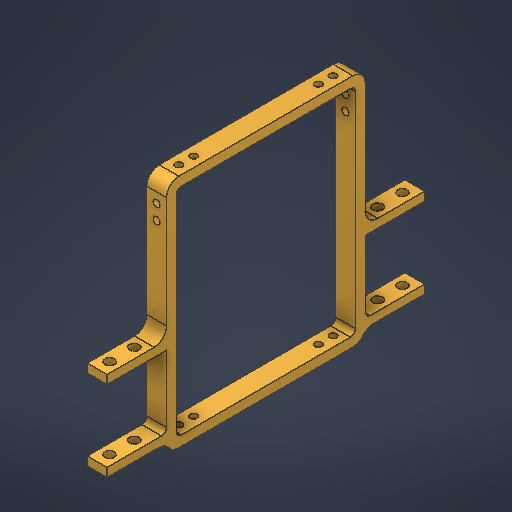
# Autodesk Inventor part: structural_ring1
Saved by Autodesk Inventor 2026.1 (Build 301233000, 233)
## iProperties
Created: 2026-05-16
Part Number: structural_ring1
Material: Generic
Document SubType Name: Modeling
Designer: emanuel
Density: 1 g/cm^3
Appearance: Default
Author: emanuel
Autodesk Inventor part; units mm, degrees
ref_plane "YZ Plane" through (0, 0, 0) normal (1, 0, 0) x (0, 1, 0)
ref_plane "XZ Plane" through (0, 0, 0) normal (0, 1, 0) x (-1, 0, 0)
ref_plane "XY Plane" through (0, 0, 0) normal (0, 0, 1) x (1, 0, 0)
sketch "Sketch1" plane through (0, 0, 0) normal (1, 0, 0) x (0, 1, 0)
  line L0 (0, 40.15) -> (0, -40.15)
  line L1 (-47.5, 0) -> (47.5, 0)
  line L2 (-47.5, 40.15) -> (47.5, 40.15)
  line L3 (47.5, 40.15) -> (47.5, -40.15)
  line L4 (47.5, -40.15) -> (-47.5, -40.15)
  line L5 (-47.5, -40.15) -> (-47.5, 40.15)
  line L6 (-47.5, 40.15) -> (47.5, -40.15) construction
  line L7 (47.5, 40.15) -> (-47.5, -40.15) construction
  line L8 (47.5, 40.15) -> (43.5, 40.15)
  line L9 (43.5, 40.15) -> (43.5, 36.15)
  line L10 (43.5, 36.15) -> (47.5, 36.15)
  line L11 (47.5, 36.15) -> (47.5, 40.15)
  line L12 (47.5, -40.15) -> (43.5, -40.15)
  line L13 (43.5, -40.15) -> (43.5, -36.15)
  line L14 (43.5, -36.15) -> (47.5, -36.15)
  line L15 (47.5, -36.15) -> (47.5, -40.15)
  line L16 (-47.5, -40.15) -> (-43.5, -40.15)
  line L17 (-43.5, -40.15) -> (-43.5, -36.15)
  line L18 (-43.5, -36.15) -> (-47.5, -36.15)
  line L19 (-47.5, -36.15) -> (-47.5, -40.15)
  line L20 (-43.5, -36.15) -> (43.5, -36.15)
  line L21 (43.5, -36.15) -> (43.5, 36.15)
  line L22 (43.5, 36.15) -> (-43.5, 36.15)
  line L23 (-43.5, 36.15) -> (-43.5, -36.15)
  point P0 (0, 0)
  dimension "d0" = 80.3
  dimension "d1" = 95
  dimension "d2" = 4
  dimension "d3" = 4
  dimension "d4" = 4
  dimension "d5" = 4
  dimension "d6" = 4
  dimension "d7" = 4
  dimension "d51" = 80.3
  constraints: 48 end point, 10 parallel, 6 horizontal, 5 perpendicular, 4 midpoint, 1 vertical
  measures "d0" distance of L0.start L0.end
  measures "d1" distance of L1.start L1.end
  measures "d2" distance of L10.end L9.end
  measures "d3" distance of L9.end L8.end
  measures "d4" distance of L13.end L14.end
  measures "d5" distance of L12.end L13.end
  measures "d6" distance of L18.end L17.end
  measures "d7" distance of L17.end L16.end
  measures "d51" distance between parallel lines of L4 L2
extrude "Extrusion1" add sketch "Sketch1" along normal blind 8 contours L2 L9 L22 L0 | L0 L22 L23 L1 L5 L2 | L2 L3 L10 L9 | L10 L3 L1 L21 | L1 L23 L18 L5 | L20 L13 L4 L0 | L0 L4 L17 L20 | L1 L3 L14 L21 | L18 L17 L4 L5 | L14 L3 L4 L13
sketch "Sketch2" plane through (8, 0, 0) normal (1, 0, 0) x (0, 0, -1)
  line L0 (40.15, 47.5) -> (-40.15, 47.5) projected
  line L1 (40.15, 47.5) -> (40.15, -10.9)
  line L2 (40.15, -47.5) -> (40.15, 47.5) projected
  line L3 (40.15, -10.9) -> (64.15, -10.9)
  line L4 (64.15, -10.9) -> (64.15, -7.4)
  line L5 (64.15, -7.4) -> (40.15, -7.4)
  line L6 (40.15, -7.4) -> (40.15, -10.9)
  line L7 (40.15, -10.9) -> (40.15, -39.9)
  line L8 (40.15, -39.9) -> (64.15, -39.9)
  line L9 (64.15, -39.9) -> (64.15, -43.4)
  line L10 (64.15, -43.4) -> (40.15, -43.4)
  line L11 (40.15, -43.4) -> (40.15, -39.9)
  line L12 (0, 47.5) -> (0, 43.5)
  line L13 (-36.15, 43.5) -> (36.15, 43.5) projected
  line L14 (-40.15, 47.5) -> (-40.15, -10.9)
  line L15 (-40.15, -47.5) -> (-40.15, 47.5)
  line L16 (-40.15, -10.9) -> (-64.15, -10.9)
  line L17 (-64.15, -10.9) -> (-64.15, -7.4)
  line L18 (-64.15, -7.4) -> (-40.15, -7.4)
  line L19 (-40.15, -7.4) -> (-40.15, -10.9)
  line L20 (-40.15, -10.9) -> (-40.15, -39.9)
  line L21 (-40.15, -39.9) -> (-64.15, -39.9)
  line L22 (-64.15, -39.9) -> (-64.15, -43.4)
  line L23 (-64.15, -43.4) -> (-40.15, -43.4)
  line L24 (-40.15, -43.4) -> (-40.15, -39.9)
  point P0 (0, 0)
  dimension "d10" = 58.4
  dimension "d11" = 24
  dimension "d12" = 3.5
  dimension "d13" = 29
  dimension "d14" = 24
  dimension "d15" = 3.5
  constraints: 44 end point, 9 symmetric about line, 4 parallel, 4 point on line, 2 horizontal, 2 midpoint, 2 perpendicular
  measures "d10" distance of L0.start L1.end
  measures "d11" distance of L5.end L4.end
  measures "d12" distance of L4.end L3.end
  measures "d13" distance of L1.end L7.end
  measures "d14" distance of L9.end L10.end
  measures "d15" distance of L8.end L9.end
extrude "Extrusion2" add sketch "Sketch2" against normal blind 8
sketch "Sketch3" plane through (8, -7.4, 64.15) normal (0, 1, 0) x (1, 0, 0)
  line L0 (0, 0) -> (-8, 0) projected
  line L1 (-4, 0) -> (-4, 5)
  line L2 (-4, 5) -> (-4, 15)
  circle A0 centre (-4, 5) radius 2
  circle A1 centre (-4, 15) radius 2
  line L3 (0, 128.3) -> (-8, 128.3) projected
  line L4 (-4, 128.3) -> (-4, 123.3)
  line L5 (-4, 123.3) -> (-4, 113.3)
  circle A2 centre (-4, 113.3) radius 2
  circle A3 centre (-4, 123.3) radius 2
  point P0 (-8, 64.15)
  dimension "d18" = 5
  dimension "d19" = 10
  dimension "d20" = 4
  dimension "d21" = 4
  dimension "d22" = 5
  dimension "d23" = 10
  dimension "d24" = 4
  dimension "d25" = 4
  constraints: 8 end point, 4 centre point, 4 coincident, 2 midpoint, 2 point on line, 2 vertical
  measures "d18" distance of L1.start L1.end
  measures "d19" distance of L1.end L2.end
  measures "d20" diameter of A0
  measures "d21" diameter of A1
  measures "d22" distance of L4.start L4.end
  measures "d23" distance of L4.end L5.end
  measures "d24" diameter of A2
  measures "d25" diameter of A3
extrude "Extrusion3" cut sketch "Sketch3" against normal blind 50
fillet "Fillet1" radius 5 4 edges at (4, 47.5, 40.15) (4, 47.5, -40.15) (4, -47.5, 40.15) (4, -47.5, -40.15)
fillet "Fillet2" radius 2 4 edges at (4, -43.5, -36.15) (4, -43.5, 36.15) (4, 43.5, 36.15) (4, 43.5, -36.15)
sketch "Sketch4" plane through (0, 47.5, 35.15) normal (0, 1, 0) x (1, 0, 0)
  line L0 (8, 0) -> (0, 0) projected
  line L1 (8, 0) -> (4, 0)
  line L2 (4, 0) -> (4, 4)
  line L3 (4, 4) -> (8, 4)
  line L4 (8, 4) -> (8, 0)
  line L5 (0, 70.3) -> (8, 70.3) projected
  line L6 (0, 70.3) -> (4, 70.3)
  line L7 (4, 70.3) -> (4, 66.3)
  line L8 (4, 66.3) -> (0, 66.3)
  line L9 (0, 66.3) -> (0, 70.3)
  line L10 (4, 66.3) -> (4, 60.3)
  line L11 (4, 4) -> (4, 10)
  circle A0 centre (4, 66.3) radius 1.45
  circle A1 centre (4, 60.3) radius 1.45
  circle A2 centre (4, 10) radius 1.45
  circle A3 centre (4, 4) radius 1.45
  point P0 (0, 35.15)
  dimension "d30" = 4
  dimension "d31" = 4
  dimension "d32" = 4
  dimension "d33" = 4
  dimension "d34" = 6
  dimension "d35" = 6
  dimension "d36" = 2.9
  dimension "d37" = 2.9
  dimension "d38" = 2.9
  dimension "d39" = 2.9
  constraints: 20 end point, 4 centre point, 4 coincident, 4 parallel, 2 horizontal, 2 perpendicular, 2 vertical
  measures "d30" distance of L2.end L3.end
  measures "d31" distance of L1.end L2.end
  measures "d32" distance of L7.end L8.end
  measures "d33" distance of L6.end L7.end
  measures "d34" distance of L7.end L10.end
  measures "d35" distance of L2.end L11.end
  measures "d36" diameter of A0
  measures "d37" diameter of A1
  measures "d38" diameter of A2
  measures "d39" diameter of A3
extrude "Extrusion4" cut sketch "Sketch4" against normal up to surface (95 mm away) contours A3 L11 L2 | L2 L3 A3 | L3 L11 A3 | A0 L10 L7 | L7 L8 A0 | L8 L10 A0 | A1 | A2
sketch "Sketch5" plane through (0, -7.4, 40.15) normal (0, 0, 1) x (1, 0, 0)
  line L0 (8, 49.9) -> (0, 49.9) projected
  line L1 (8, 49.9) -> (4, 49.9)
  line L2 (4, 49.9) -> (4, 45.9)
  line L3 (4, 45.9) -> (8, 45.9)
  line L4 (8, 45.9) -> (8, 49.9)
  line L5 (4, 45.9) -> (4, 39.9)
  circle A0 centre (4, 45.9) radius 1.45
  circle A1 centre (4, 39.9) radius 1.45
  point P0 (0, 7.4)
  dimension "d42" = 4
  dimension "d43" = 4
  dimension "d44" = 6
  dimension "d45" = 2.9
  dimension "d46" = 2.9
  constraints: 10 end point, 2 centre point, 2 coincident, 2 parallel, 1 horizontal, 1 perpendicular, 1 vertical
  measures "d42" distance of L3.end L2.end
  measures "d43" distance of L2.end L1.end
  measures "d44" distance of L2.end L5.end
  measures "d45" diameter of A0
  measures "d46" diameter of A1
extrude "Extrusion5" cut sketch "Sketch5" against normal up to surface (80.3 mm away) contours A0 L3 L2 | L2 L5 A0 | A0 L5 L3 | A1
fillet "Fillet3" radius 5 4 edges at (4, -7.4, -40.15) (4, -7.4, 40.15) (4, -43.4, 40.15) (4, -43.4, -40.15)
fillet "Fillet4" radius 2 2 edges at (4, -39.9, 40.15) (4, -39.9, -40.15)
body "Solid1"
